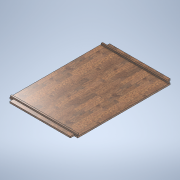
# Autodesk Inventor part: tub floor 2
Saved by Autodesk Inventor 2020 (Build 240168000, 168)
## iProperties
Created: 2020-06-26
Part Number: tub floor 2
Material: Generic
Document SubType Name: Modeling
Designer: Abbas
Density: 1 g/cm^3
Appearance: Default
Author: Abbas
Autodesk Inventor part; units mm, degrees
ref_plane "YZ Plane" through (0, 0, 0) normal (1, 0, 0) x (0, 1, 0)
ref_plane "XZ Plane" through (0, 0, 0) normal (0, 1, 0) x (-1, 0, 0)
ref_plane "XY Plane" through (0, 0, 0) normal (0, 0, 1) x (1, 0, 0)
sketch "Sketch1" plane through (0, 0, 0) normal (0, 1, 0) x (-1, 0, 0)
  line L0 (408.912, 674) -> (-408.912, 674)
  line L1 (-458.912, 624) -> (-458.912, -624)
  line L2 (-408.912, -674) -> (408.912, -674)
  line L3 (458.912, -624) -> (458.912, 624)
  line L4 (458.912, 674) -> (-458.912, -674) construction
  line L5 (408.912, 674) -> (408.912, 624)
  line L6 (408.912, 624) -> (458.912, 624)
  line L7 (458.912, 674) -> (408.912, 624) construction
  line L8 (408.912, 674) -> (458.912, 624) construction
  line L9 (-458.912, 624) -> (-408.912, 624)
  line L10 (-408.912, 624) -> (-408.912, 674)
  line L11 (-408.912, 674) -> (-458.912, 624) construction
  line L12 (-458.912, 674) -> (-408.912, 624) construction
  line L13 (458.912, -624) -> (408.912, -624)
  line L14 (408.912, -624) -> (408.912, -674)
  line L15 (458.912, -624) -> (408.912, -674) construction
  line L16 (408.912, -624) -> (458.912, -674) construction
  line L17 (-408.912, -624) -> (-458.912, -624)
  line L18 (-408.912, -674) -> (-408.912, -624)
  line L19 (-408.912, -624) -> (-458.912, -674) construction
  line L20 (-458.912, -624) -> (-408.912, -674) construction
  point P0 (0, 0)
  point P1 (433.912, 649)
  point P2 (-433.912, 649)
  point P3 (433.912, -649)
  point P4 (-433.912, -649)
  constraints: 42 end point, 9 midpoint, 3 horizontal, 2 parallel, 2 perpendicular
extrude "Extrusion1" add sketch "Sketch1" along normal blind 20
sketch "Sketch2" plane through (0, 20, 0) normal (0, 1, 0) x (1, 0, 0)
  line L0 (452, 602) -> (-452, 602)
  line L1 (-452, -602) -> (452, -602)
  line L2 (452, 602) -> (-452, -602) construction
  line L3 (-452, 602) -> (452, -602) construction
  line L4 (452, 622) -> (-452, 622)
  line L5 (-452, -622) -> (452, -622)
  line L6 (452, 622) -> (-452, -622) construction
  line L7 (-452, 622) -> (452, -622) construction
  line L8 (452, -622) -> (452, -602)
  line L9 (452, 602) -> (452, 622)
  line L10 (-452, 622) -> (-452, 602)
  line L11 (-452, -602) -> (-452, -622)
  point P0 (0, 0)
  constraints: 24 end point, 6 parallel, 4 midpoint, 2 horizontal, 2 perpendicular
extrude "Extrusion2" add sketch "Sketch2" along normal blind 20
body "Solid1"
